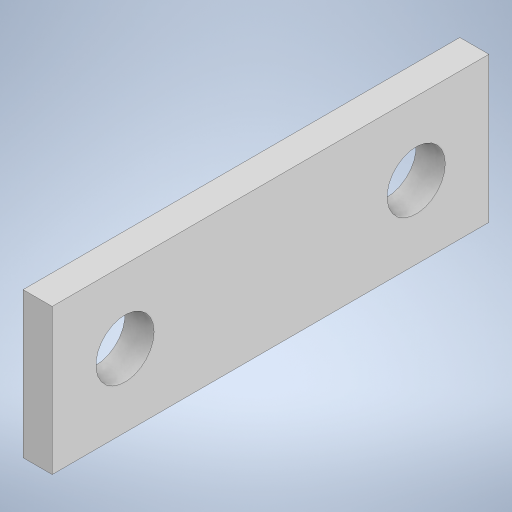
# Autodesk Inventor part: Pengunci sendok
Saved by Autodesk Inventor 2024 (Build 280153000, 153)
## iProperties
Created: 2023-10-30
Part Number: Pengunci sendok
Material: Generic
Document SubType Name: Modeling
Designer: lazy1
Density: 1 g/cm^3
Appearance: Default
Author: lazy1
Autodesk Inventor part; units mm, degrees
ref_plane "YZ Plane" through (0, 0, 0) normal (1, 0, 0) x (0, 1, 0)
ref_plane "XZ Plane" through (0, 0, 0) normal (0, 1, 0) x (-1, 0, 0)
ref_plane "XY Plane" through (0, 0, 0) normal (0, 0, 1) x (1, 0, 0)
sketch "Sketch1" plane through (0, 0, 0) normal (0, 1, 0) x (-1, 0, 0)
  line L0 (-1, 15) -> (1, 15)
  line L1 (1, 15) -> (1, -15)
  line L2 (1, -15) -> (-1, -15)
  line L3 (-1, -15) -> (-1, 15)
  line L4 (-1, 15) -> (1, -15) construction
  line L5 (1, 15) -> (-1, -15) construction
  point P0 (0, 0)
  dimension "d0" = 2
  dimension "d1" = 30
  constraints: 12 end point, 2 midpoint, 2 parallel, 1 horizontal, 1 perpendicular
  measures "d0" distance of L1.end L2.end
  measures "d1" distance of L0.end L1.end
extrude "Extrusion1" add sketch "Sketch1" along normal blind 10
sketch "Sketch3" plane through (1, 0, 15) normal (1, 0, 0) x (0, 0, -1)
  line L0 (0, 0) -> (0, 10) projected
  line L1 (0, 5) -> (5, 5)
  line L2 (30, 0) -> (30, 10) projected
  line L3 (30, 5) -> (25, 5)
  point P0 (15, 0)
  dimension "d13" = 5
  dimension "d14" = 5
  constraints: 4 end point, 2 coincident, 2 horizontal, 2 midpoint
  measures "d13" distance of L1.start L1.end
  measures "d14" distance of L3.start L3.end
hole "Hole2" at (1, 5, 10) at (1, 5, -10) direction (-1, 0, 0) diameter 4 depth 8 tip angle 118
body "Solid1"
